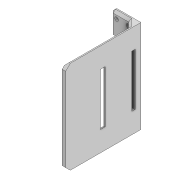
# Autodesk Inventor part: patas
Saved by Autodesk Inventor 2022 (Build 260153000, 153)
## iProperties
Created: 2022-11-19
Part Number: patas
Material: Genérico
Document SubType Name: Modeling
Designer: Jorge
Density: 1 g/cm^3
Appearance: Valor por defecto
Author: Jorge
Autodesk Inventor part; units mm, degrees
ref_plane "YZ Plane" through (0, 0, 0) normal (1, 0, 0) x (0, 1, 0)
ref_plane "XZ Plane" through (0, 0, 0) normal (0, 1, 0) x (-1, 0, 0)
ref_plane "XY Plane" through (0, 0, 0) normal (0, 0, 1) x (1, 0, 0)
sketch "Boceto1" plane through (0, 0, 0) normal (0, 0, 1) x (1, 0, 0)
  line L0 (0, 0) -> (20, 0)
  line L1 (20, 0) -> (20, 80)
  line L2 (20, 80) -> (0, 80)
  line L3 (0, 80) -> (0, 0)
  dimension "d0" = 20
  dimension "d1" = 80
  constraints: 8 end point, 2 parallel, 1 horizontal, 1 perpendicular
  measures "d0" distance of L2.end L1.end
  measures "d1" distance of L1.end L0.end
extrude "Extrusión1" add sketch "Boceto1" along normal blind 3
sketch "Boceto2" plane through (0, 0, 3) normal (0, 0, 1) x (1, 0, 0)
  line L0 (20, 0) -> (20, 80) construction
  line L1 (20, 80) -> (0, 80) construction
  line L2 (0, 80) -> (0, 0) construction
  line L3 (0, 0) -> (20, 0) construction
  line L4 (0, 80) -> (0, 0) construction
  line L5 (0, 75) -> (20, 75) construction
  line L6 (20, 0) -> (20, 80) construction
  line L7 (20, 80) -> (0, 80) construction
  line L8 (15, 80) -> (15, 0) construction
  line L9 (0, 0) -> (20, 0) construction
  line L10 (0, 5) -> (20, 5) construction
  circle A0 centre (15, 5) radius 1.6
  circle A1 centre (15, 75) radius 1.6
  line L11 (0, 65) -> (20, 65) construction
  line L12 (0, 15) -> (20, 15) construction
  line L13 (5, 80) -> (5, 0) construction
  circle A2 centre (15, 65) radius 1.6
  circle A3 centre (5, 75) radius 1.6
  circle A4 centre (5, 5) radius 1.6
  circle A5 centre (15, 15) radius 1.6
  line L14 (10, 80) -> (10, 0) construction
  line L15 (0, 40) -> (20, 40) construction
  dimension "d4" = 3.2
  dimension "d7" = 3.2
  dimension "d9" = 3.2
  dimension "d10" = 3.2
  dimension "d11" = 3.2
  dimension "d12" = 3.2
  dimension "d13" = 10
  dimension "d14" = 10
  dimension "d15" = 10
  dimension "d16" = 5
  dimension "d17" = 70
  dimension "d18" = 35
  constraints: 24 point on line, 16 end point, 6 centre point, 6 perpendicular, 4 midpoint
  measures "d4" diameter of A0
  measures "d7" diameter of A1
  measures "d9" diameter of A2
  measures "d10" diameter of A3
  measures "d11" diameter of A4
  measures "d12" diameter of A5
  measures "d13" distance between parallel lines of L8 L13
  measures "d14" distance between parallel lines of L11 L5
  measures "d15" distance between parallel lines of L10 L12
  measures "d16" distance between parallel lines of L14 L13
  measures "d17" distance between parallel lines of L10 L5
  measures "d18" distance between parallel lines of L15 L5
extrude "Extrusión2" cut sketch "Boceto2" against normal through all
sketch "Boceto3" plane through (0, 0, 3) normal (0, 0, 1) x (1, 0, 0)
  circle A0 centre (5, 75) radius 1.6 projected
  circle A1 centre (15, 5) radius 1.6 projected
  circle A2 centre (15, 65) radius 1.6 projected
  circle A3 centre (15, 75) radius 1.6 projected
  circle A4 centre (5, 5) radius 1.6 projected
  circle A5 centre (15, 15) radius 1.6 projected
  line L0 (20, 0) -> (20, 80) projected
  line L1 (20, 80) -> (0, 80) projected
  line L2 (0, 80) -> (0, 0) projected
  line L3 (0, 0) -> (20, 0) projected
  line L4 (0, 80) -> (0, 0) projected
  line L5 (0, 60) -> (7.8934, 60)
  line L6 (7.8934, 60) -> (15, 55)
  line L7 (15, 25) -> (11.4821, 20)
  line L8 (11.4821, 20) -> (0, 20)
  line L9 (15, 55) -> (15, 25)
  line L10 (0, 40) -> (20, 40) construction
  line L11 (20, 0) -> (20, 80) construction
  line L12 (0, 60) -> (0, 20)
  dimension "d21" = 20
  dimension "d22" = 20
  dimension "d23" = 30
  dimension "d24" = 15
  dimension "d26" = 5
  constraints: 14 end point, 3 perpendicular, 2 midpoint, 2 point on line, 1 horizontal, 1 vertical
  measures "d21" distance between parallel lines of L1 L5
  measures "d22" distance between parallel lines of L3 L8
  measures "d23" distance of L6.end L7.start
  measures "d24" distance from line of L10 L6.end
  measures "d26" distance between parallel lines of L9 L0
extrude "Extrusión3" cut sketch "Boceto3" against normal through all contours L2 L5 L6 L9 L7 L8
sketch "Boceto5" plane through (0, 0, 0) normal (0, 0, -1) x (-1, 0, 0)
  line L0 (0, 20) -> (-11.4821, 20) construction
  line L1 (-11.4821, 20) -> (-15, 25) construction
  line L2 (-15, 25) -> (-15, 55) construction
  line L3 (-15, 55) -> (-7.8934, 60) construction
  line L4 (-7.8934, 60) -> (0, 60) construction
  line L5 (0, 80) -> (0, 60) construction
  line L6 (-20, 80) -> (0, 80) construction
  line L7 (-20, 0) -> (-20, 80) construction
  line L8 (0, 0) -> (-20, 0) construction
  line L9 (0, 20) -> (0, 0) construction
  circle A0 centre (-15, 15) radius 1.6 construction
  circle A1 centre (-5, 5) radius 1.6 construction
  circle A2 centre (-15, 75) radius 1.6 construction
  circle A3 centre (-15, 65) radius 1.6 construction
  circle A4 centre (-15, 5) radius 1.6 construction
  circle A5 centre (-5, 75) radius 1.6 construction
  line L10 (-20, 80) -> (-23, 80)
  line L11 (-23, 80) -> (-23, 0)
  line L12 (-23, 0) -> (-20, 0)
  line L13 (-20, 0) -> (-20, 80)
  dimension "d29" = 3
  constraints: 8 end point, 2 parallel, 1 horizontal, 1 perpendicular
  measures "d29" distance of L12.end L11.end
extrude "Extrusión4" add sketch "Boceto5" against normal blind 35
sketch "Boceto6" plane through (20, 0, 3) normal (-1, 0, 0) x (0, 0, 1)
  line L0 (0, 0) -> (0, 80) construction
  line L1 (0, 0) -> (32, 0) construction
  line L2 (32, 80) -> (32, 0) construction
  line L3 (0, 80) -> (32, 80) construction
  line L4 (0, 80) -> (32, 80) construction
  line L5 (2, 80) -> (2, 0) construction
  line L6 (0, 0) -> (32, 0) construction
  line L7 (2, 62.5) -> (5, 62.5)
  line L8 (5, 62.5) -> (5, 17.5)
  line L9 (5, 17.5) -> (2, 17.5)
  line L10 (2, 17.5) -> (2, 62.5)
  line L11 (0, 55) -> (0, 25) construction
  line L12 (0, 40) -> (32, 40) construction
  line L13 (32, 80) -> (32, 0) construction
  line L14 (29.5, 80) -> (29.5, 0) construction
  line L15 (3.5, 62.5) -> (3.5, 80) construction
  line L16 (28, 62.5) -> (31, 62.5)
  line L17 (31, 62.5) -> (31, 17.5)
  line L18 (31, 17.5) -> (28, 17.5)
  line L19 (28, 17.5) -> (28, 62.5)
  line L20 (31, 62.5) -> (32, 62.5)
  line L21 (32, 62.5) -> (32, 17.5)
  line L22 (32, 17.5) -> (31, 17.5)
  line L23 (31, 17.5) -> (31, 62.5)
  point P0 (-3, 0)
  point P1 (31, 17.5)
  dimension "d32" = 2
  dimension "d33" = 3
  dimension "d34" = 45
  dimension "d35" = 22.5
  dimension "d37" = 26
  dimension "d38" = 3
  dimension "d39" = 1.5
  constraints: 32 end point, 7 point on line, 6 parallel, 6 perpendicular, 3 horizontal, 3 midpoint
  measures "d32" distance between parallel lines of L0 L5
  measures "d33" distance of L8.end L9.end
  measures "d34" distance of L7.end L8.end
  measures "d35" distance between parallel lines of L12 L7
  measures "d37" distance between parallel lines of L15 L14
  measures "d38" distance of L17.end L18.end
  measures "d39" distance between parallel lines of L14 L19
extrude "Extrusión5" cut sketch "Boceto6" against normal through all
chamfer "Chaflán1" distance 4.9 angle 45 1 edges at (20, 40, 3)
sketch "Boceto7" plane through (0, 0, 3) normal (0, 0, 1) x (1, 0, 0)
  arc A0 (15.1, 16.5969) -> (15.1, 13.4031) centre (15, 15) ccw construction
  arc A1 (15.1, 6.5969) -> (15.1, 3.4031) centre (15, 5) ccw construction
  arc A2 (15.1, 66.5969) -> (15.1, 63.4031) centre (15, 65) ccw construction
  arc A3 (15.1, 76.5969) -> (15.1, 73.4031) centre (15, 75) ccw construction
  circle A4 centre (15, 75) radius 3.5
  circle A5 centre (15, 65) radius 1.6 projected
  circle A6 centre (15, 65) radius 3.5
  circle A7 centre (15, 15) radius 3.5
  circle A8 centre (15, 5) radius 1.6 projected
  circle A9 centre (15, 5) radius 3.5
  point P0 (0, 0)
  dimension "d45" = 7
  dimension "d46" = 7
  dimension "d47" = 7
  dimension "d48" = 7
  constraints: 4 centre point, 4 coincident
  measures "d45" diameter of A4
  measures "d46" diameter of A6
  measures "d47" diameter of A7
  measures "d48" diameter of A9
extrude "Extrusión6" cut sketch "Boceto7" along normal blind 10 contours A4 | A5 | A6 | A7 | A8 | A9
sketch "Boceto8" plane through (20, 17.5, 8) normal (-1, 0, 0) x (0, 0, 1)
  line L0 (27, 62.5) -> (27, 45) projected
  line L1 (27, 62.5) -> (57, 62.5)
  line L2 (57, 62.5) -> (57, -17.5)
  line L3 (57, -17.5) -> (27, -17.5)
  line L4 (27, -17.5) -> (27, 62.5)
  point P0 (-8, -17.5)
  dimension "d57" = 30
  constraints: 8 end point, 2 parallel, 1 horizontal, 1 perpendicular
  measures "d57" distance of L2.end L3.end
extrude "Extrusión7" add sketch "Boceto8" against normal blind 3
chamfer "Chaflán4" distance 4 angle 45 2 edges at (21.5, 0, 65) (21.5, 80, 65)
chamfer "Chaflán5" distance 2 angle 45 22 edges at (7.55, 80, 3) (0, 70, 3) (0, 80, 1.5) (0, 60, 1.5) (3.9467, 60, 3) (11.4467, 57.5, 3) (13.2411, 22.5, 3) (5.7411, 20, 3) (0, 10, 3) (7.55, 0, 3) (0, 20, 1.5) (0, 0, 1.5) (17.55, 80, 5.45) (17.55, 0, 5.45) (20, 0, 34.45) (20, 80, 34.45) (20, 40, 35) (20, 40, 31) (20, 62.5, 33) (20, 17.5, 33) (20, 40, 8) (17.1, 40, 5)
equation "\"d16\" = 0.5 * d13"
equation "\"d18\" = 0.5 * d17"
equation "\"d24\" = 0.5 * d23"
equation "\"d35\" = 0.5 * d34"
equation "\"d39\" = 0.5 * d38"
